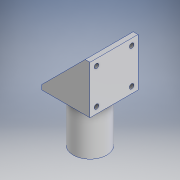
# Autodesk Inventor part: motormount
Saved by Autodesk Inventor 2016 (Build 200138000, 138)
## iProperties
Created: 2017-05-27
Part Number: motormount
Material: Aluminum 6061
Document SubType Name: Modeling
Designer: Kyle
Density: 2.7 g/cm^3
Appearance: Aluminum - Flat
Mass: 41.2941 g
Surface Area: 92.7958 cm^2
Volume: 15.2941 cm^3
Author: Kyle
Autodesk Inventor part; units mm, degrees
ref_plane "YZ Plane" through (0, 0, 0) normal (1, 0, 0) x (0, 1, 0)
ref_plane "XZ Plane" through (0, 0, 0) normal (0, 1, 0) x (-1, 0, 0)
ref_plane "XY Plane" through (0, 0, 0) normal (0, 0, 1) x (1, 0, 0)
sketch "Sketch2" plane through (0, 0, 0) normal (0, 1, 0) x (-1, 0, 0)
  line L0 (0, 0) -> (31.75, 0)
  line L1 (31.75, 0) -> (31.75, -31.75)
  line L2 (31.75, -31.75) -> (0, -31.75)
  line L3 (0, -31.75) -> (0, 0)
  dimension "d0" = 31.75
  dimension "d1" = 31.75
  constraints: 8 end point, 2 parallel, 1 horizontal, 1 perpendicular
  measures "d0" distance of L1.end L2.end
  measures "d1" distance of L0.end L1.end
extrude "Extrusion1" add sketch "Sketch2" along normal blind 31.75
sketch "Sketch3" plane through (-31.75, 0, 0) normal (0, 0, 1) x (1, 0, 0)
  line L0 (0, 31.75) -> (31.75, 31.75) projected
  line L1 (28.575, 31.75) -> (0, 3.175)
  line L2 (0, 0) -> (0, 31.75) projected
  line L3 (28.575, 31.75) -> (68.9862, 31.75) construction
  line L4 (0, 0) -> (0, 31.75) projected
  line L5 (0, 31.75) -> (14.2875, 17.4625) construction
  point P0 (31.75, 0)
  dimension "d4" = 135
  dimension "d25" = 3.175
  dimension "d26" = 20.2056
  constraints: 6 end point, 2 point on line, 1 equal length, 1 horizontal, 1 midpoint
  measures "d4" angle of L1 L3
  measures "d25" distance of L0.end L1.start
  measures "d26" distance of L0.start L5.end
extrude "Extrusion2" cut sketch "Sketch3" against normal blind 38.1
sketch "Sketch4" plane through (0, 0, 0) normal (0, -1, 0) x (1, 0, 0)
  line L0 (-31.75, 0) -> (0, -31.75) construction
  circle A0 centre (-15.875, -15.875) radius 11.0808
  point P0 (0, 0)
  dimension "d7" = 22.1615
  constraints: 2 coincident, 2 end point, 1 centre point, 1 midpoint
  measures "d7" diameter of A0
extrude "Extrusion3" add sketch "Sketch4" along normal blind 31.75
sketch "Sketch5" plane through (-15.875, -31.75, -15.875) normal (0, -1, 0) x (1, 0, 0)
  circle A0 centre (0, 0) radius 8.7313
  circle A1 centre (0, 0) radius 11.0808 projected
  point P0 (15.875, 15.875)
  dimension "d35" = 17.4625
  constraints: 1 centre point, 1 coincident
  measures "d35" diameter of A0
extrude "Extrusion4" cut sketch "Sketch5" against normal through all contours A0
sketch "Sketch6" plane through (0, 0, 0) normal (1, 0, 0) x (0, 0, -1)
  line L0 (0, 31.75) -> (31.75, 0) construction
  line L1 (4.2545, 4.2545) -> (27.4955, 4.2545) construction
  line L2 (27.4955, 4.2545) -> (27.4955, 27.4955) construction
  line L3 (27.4955, 27.4955) -> (4.2545, 27.4955) construction
  line L4 (4.2545, 27.4955) -> (4.2545, 4.2545) construction
  line L5 (4.2545, 4.2545) -> (27.4955, 27.4955) construction
  line L6 (27.4955, 4.2545) -> (4.2545, 27.4955) construction
  circle A0 centre (4.2545, 27.4955) radius 1.5
  circle A1 centre (4.2545, 4.2545) radius 1.5
  circle A2 centre (27.4955, 4.2545) radius 1.5
  circle A3 centre (27.4955, 27.4955) radius 1.5
  line L7 (0, 31.75) -> (31.75, 31.75) projected
  point P0 (0, 0)
  point P1 (15.875, 15.875)
  dimension "d15" = 23.241
  dimension "d16" = 23.241
  dimension "d17" = 3
  dimension "d20" = 360
  dimension "d24" = 4.2545
  constraints: 14 end point, 4 centre point, 3 coincident, 3 midpoint, 2 parallel, 1 horizontal, 1 perpendicular, 9 other
  measures "d15" distance of L3.end L2.end
  measures "d16" distance of L2.end L1.end
  measures "d17" diameter of A0
  measures "d24" distance between parallel lines of L7 L3
extrude "Extrusion5" cut sketch "Sketch6" against normal blind 12.7
thread "Thread1" size "M3x0.5" class "6H" standard "ANSI Metric M Profile" full length
thread "Thread2" size "M3x0.5" class "6H" standard "ANSI Metric M Profile" full length
thread "Thread3" size "M3x0.5" class "6H" standard "ANSI Metric M Profile" full length
thread "Thread4" size "M3x0.5" class "6H" standard "ANSI Metric M Profile" full length
body "Solid1"
